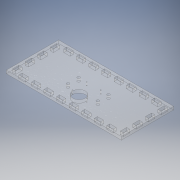
# Autodesk Inventor part: case_top
Saved by Autodesk Inventor 2019 (Build 230136000, 136)
## iProperties
Created: 2019-02-02
Part Number: case_top
Material: Acrylic, Clear
Document SubType Name: Modeling
Designer: suchanek
Density: 1.19 g/cm^3
Appearance: Transparent - Clear
Author: suchanek
Autodesk Inventor part; units mm, degrees
ref_plane "YZ Plane" through (0, 0, 0) normal (1, 0, 0) x (0, 1, 0)
ref_plane "XZ Plane" through (0, 0, 0) normal (0, 1, 0) x (-1, 0, 0)
ref_plane "XY Plane" through (0, 0, 0) normal (0, 0, 1) x (1, 0, 0)
sketch "Sketch1" plane through (0, 0, 0) normal (0, 1, 0) x (-1, 0, 0)
  line L0 (110, 50) -> (-110, 50)
  line L1 (-110, 50) -> (-110, -50)
  line L2 (-110, -50) -> (110, -50)
  line L3 (110, -50) -> (110, 50)
  line L4 (110, 50) -> (-110, -50) construction
  line L5 (-110, 50) -> (110, -50) construction
  circle A0 centre (-13.5, 20) radius 0.9
  circle A1 centre (13.5, 20) radius 0.9
  circle A2 centre (13.5, -7) radius 0.9
  circle A3 centre (-13.5, -7) radius 0.9
  line L6 (-13.5, 20) -> (13.5, 20)
  line L7 (13.5, -7) -> (-13.5, -7)
  line L8 (0, 0) -> (4.5236, 0)
  circle A4 centre (28.5, -7) radius 2.6
  circle A5 centre (-28.5, -7) radius 2.6
  circle A6 centre (28.5, 13.5) radius 2.6
  circle A7 centre (-28.5, 13.5) radius 2.6
  line L9 (0, -7) -> (0, -18)
  line L10 (0, 0) -> (5.2635, 0)
  line L11 (106, -42) -> (100, -42)
  line L12 (100, -42) -> (100, -30)
  line L13 (100, -30) -> (106, -30)
  line L14 (106, -30) -> (106, -42)
  line L15 (106, -18) -> (100, -18)
  line L16 (100, -18) -> (100, -6)
  line L17 (100, -6) -> (106, -6)
  line L18 (106, -6) -> (106, -18)
  line L19 (66, -40) -> (54, -40)
  line L20 (54, -40) -> (54, -46)
  line L21 (54, -46) -> (66, -46)
  line L22 (66, -46) -> (66, -40)
  line L23 (42, -40) -> (30, -40)
  line L24 (30, -40) -> (30, -46)
  line L25 (30, -46) -> (42, -46)
  line L26 (42, -46) -> (42, -40)
  line L27 (18, -40) -> (6, -40)
  line L28 (6, -40) -> (6, -46)
  line L29 (6, -46) -> (18, -46)
  line L30 (18, -46) -> (18, -40)
  line L31 (78, -46) -> (90, -46)
  line L32 (90, -46) -> (90, -40)
  line L33 (90, -40) -> (78, -40)
  line L34 (78, -40) -> (78, -46)
  line L35 (-106, -42) -> (-100, -42)
  line L36 (-100, -42) -> (-100, -30)
  line L37 (-100, -30) -> (-106, -30)
  line L38 (-106, -30) -> (-106, -42)
  line L39 (-106, -18) -> (-100, -18)
  line L40 (-100, -18) -> (-100, -6)
  line L41 (-100, -6) -> (-106, -6)
  line L42 (-106, -6) -> (-106, -18)
  line L43 (-66, -40) -> (-54, -40)
  line L44 (-54, -40) -> (-54, -46)
  line L45 (-54, -46) -> (-66, -46)
  line L46 (-66, -46) -> (-66, -40)
  line L47 (-42, -40) -> (-30, -40)
  line L48 (-30, -40) -> (-30, -46)
  line L49 (-30, -46) -> (-42, -46)
  line L50 (-42, -46) -> (-42, -40)
  line L51 (-18, -40) -> (-6, -40)
  line L52 (-6, -40) -> (-6, -46)
  line L53 (-6, -46) -> (-18, -46)
  line L54 (-18, -46) -> (-18, -40)
  line L55 (-78, -46) -> (-90, -46)
  line L56 (-90, -46) -> (-90, -40)
  line L57 (-90, -40) -> (-78, -40)
  line L58 (-78, -40) -> (-78, -46)
  line L59 (106, 42) -> (100, 42)
  line L60 (100, 42) -> (100, 30)
  line L61 (100, 30) -> (106, 30)
  line L62 (106, 30) -> (106, 42)
  line L63 (106, 18) -> (100, 18)
  line L64 (100, 18) -> (100, 6)
  line L65 (100, 6) -> (106, 6)
  line L66 (106, 6) -> (106, 18)
  line L67 (66, 40) -> (54, 40)
  line L68 (54, 40) -> (54, 46)
  line L69 (54, 46) -> (66, 46)
  line L70 (66, 46) -> (66, 40)
  line L71 (42, 40) -> (30, 40)
  line L72 (30, 40) -> (30, 46)
  line L73 (30, 46) -> (42, 46)
  line L74 (42, 46) -> (42, 40)
  line L75 (18, 40) -> (6, 40)
  line L76 (6, 40) -> (6, 46)
  line L77 (6, 46) -> (18, 46)
  line L78 (18, 46) -> (18, 40)
  line L79 (78, 46) -> (90, 46)
  line L80 (90, 46) -> (90, 40)
  line L81 (90, 40) -> (78, 40)
  line L82 (78, 40) -> (78, 46)
  line L83 (-100, 30) -> (-106, 30)
  line L84 (-106, 18) -> (-100, 18)
  line L85 (-100, 18) -> (-100, 6)
  line L86 (-100, 6) -> (-106, 6)
  line L87 (-106, 6) -> (-106, 18)
  line L88 (-106, 42) -> (-100, 42)
  line L89 (-106, 30) -> (-106, 42)
  line L90 (-100, 42) -> (-100, 30)
  line L91 (-90, 40) -> (-78, 40)
  line L92 (-90, 46) -> (-90, 40)
  line L93 (-78, 46) -> (-90, 46)
  line L94 (-78, 40) -> (-78, 46)
  line L95 (-66, 46) -> (-66, 40)
  line L96 (-54, 40) -> (-54, 46)
  line L97 (-54, 46) -> (-66, 46)
  line L98 (-66, 40) -> (-54, 40)
  line L99 (-6, 40) -> (-6, 46)
  line L100 (-18, 40) -> (-6, 40)
  line L101 (-6, 46) -> (-18, 46)
  line L102 (-18, 46) -> (-18, 40)
  line L103 (-30, 40) -> (-30, 46)
  line L104 (-42, 46) -> (-42, 40)
  line L105 (-30, 46) -> (-42, 46)
  line L106 (-42, 40) -> (-30, 40)
  circle A8 centre (0, 21) radius 12
  point P0 (0, 0)
  point P1 (0, 0)
  point P2 (11.5, -7)
  point P3 (-11.5, -7)
  dimension "d0" = 100
  dimension "d1" = 220
  dimension "d2" = 27
  dimension "d3" = 1.8
  dimension "d4" = 5.2
  dimension "d5" = 15
  dimension "d6" = 27
  dimension "d31" = 6
  dimension "d32" = 4
  dimension "d34" = 6
  dimension "d35" = 12
  dimension "d36" = 12
  dimension "d37" = 12
  dimension "d38" = 6
  dimension "d39" = 12
  dimension "d40" = 12
  dimension "d41" = 12
  dimension "d42" = 12
  dimension "d43" = 12
  dimension "d44" = 12
  dimension "d45" = 12
  dimension "d46" = 6
  dimension "d47" = 4
  dimension "d50" = 2
  dimension "d53" = 20.5
  dimension "d54" = 20
  dimension "d56" = 24
  dimension "d57" = 1
  constraints: 214 end point, 73 symmetric about line, 23 point on line, 14 parallel, 11 horizontal, 9 centre point, 7 midpoint, 7 perpendicular, 6 equal radius, 5 vertical alignment, 3 collinear, 3 horizontal alignment, 1 vertical
  measures "d0" distance of L2.end L0.start
  measures "d1" distance of L1.end L2.end
  measures "d2" distance of L7.start L6.end
  measures "d3" diameter of A2
  measures "d4" diameter of A5
  measures "d5" distance of A5.centre L7.end
  measures "d6" distance of L7.start L7.end
  measures "d31" distance between parallel lines of L16 L18
  measures "d32" distance between parallel lines of L3 L18
  measures "d34" distance between parallel lines of L17 L10
  measures "d35" distance of L17.end L15.start
  measures "d36" distance between parallel lines of L15 L13
  measures "d37" distance of L13.end L11.start
  measures "d38" distance between parallel lines of L28 L9
  measures "d39" distance of L28.end L29.end
  measures "d40" distance between parallel lines of L30 L24
  measures "d41" distance of L23.start L23.end
  measures "d42" distance between parallel lines of L26 L20
  measures "d43" distance of L19.start L19.end
  measures "d44" distance between parallel lines of L22 L34
  measures "d45" distance of L32.end L33.end
  measures "d46" distance of L27.end L28.end
  measures "d47" distance between parallel lines of L2 L29
  measures "d50" distance of point (-11.5, -7) L7.end
  measures "d53" distance of A4.centre A6.centre
  measures "d54" distance between parallel lines of L6 L8
  measures "d56" diameter of A8
  measures "d57" distance from line of L6 A8.centre
extrude "Extrusion3" add sketch "Sketch1" along normal blind 6
body "Solid3"
